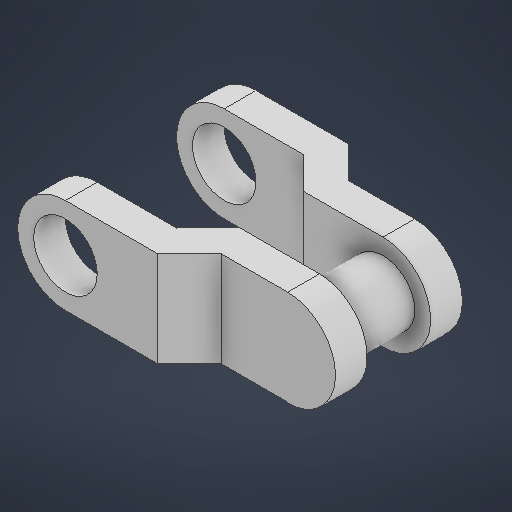
# Autodesk Inventor part: Pieza2
Saved by Autodesk Inventor 2026.2 (Build 302298010, 298A)
## iProperties
Created: 2026-03-27
Part Number: Pieza2
Material: Genérico
Document SubType Name: Modeling
Designer: agusb
Density: 1 g/cm^3
Appearance: Valor por defecto
Author: agusb
Autodesk Inventor part; units mm, degrees
ref_plane "YZ Plane" through (0, 0, 0) normal (1, 0, 0) x (0, 1, 0)
ref_plane "XZ Plane" through (0, 0, 0) normal (0, 1, 0) x (-1, 0, 0)
ref_plane "XY Plane" through (0, 0, 0) normal (0, 0, 1) x (1, 0, 0)
sketch "Boceto1" plane through (0, 0, 0) normal (0, 1, 0) x (-1, 0, 0)
  line L0 (0, -10) -> (44.14, -10)
  line L1 (44.14, -10) -> (44.14, 0)
  line L2 (44.14, 0) -> (4.14, 0)
  line L3 (4.14, 0) -> (14.14, 0) construction
  line L4 (4.14, 0) -> (14.14, 0) construction
  line L5 (-5.86, 10) -> (4.14, 0)
  line L6 (-10, 0) -> (0, -10)
  line L7 (-10, 0) -> (-45.86, 0)
  line L8 (-10, 0) -> (25.86, 0) construction
  line L9 (-45.86, 0) -> (-45.86, 10)
  line L10 (-45.86, 10) -> (-5.86, 10)
  point P0 (0, 0)
  dimension "d10" = 44.14
  dimension "d12" = 40
  dimension "d19" = 35.86
  dimension "d21" = 10
  constraints: 22 end point, 5 horizontal, 2 perpendicular, 1 collinear, 1 vertical
  measures "d10" distance of L0.start L0.end
  measures "d12" distance of L1.end L2.end
  measures "d19" distance of L6.start L7.end
  measures "d21" distance of L7.end L9.end
extrude "Extrusión1" add sketch "Boceto1" along normal blind 30
sketch "Boceto2" plane through (5.86, 0, 10) normal (0, 0, 1) x (1, 0, 0)
  point P0 (-5.86, 0)
sketch "Boceto3" plane through (0, 0, -10) normal (0, 0, -1) x (-1, 0, 0)
  line L0 (44.14, 0) -> (44.14, 30) projected
  line L1 (0, 0) -> (0, 30) projected
  line L2 (44.14, 0) -> (44.14, 15)
  line L3 (44.14, 0) -> (59.14, 0) construction
  circle A0 centre (29.14, 15) radius 10
  line L4 (0, 0) -> (44.14, 0) projected
  line L5 (29.14, 15) -> (44.14, 15) construction
  arc A1 (29.14, 0) -> (29.14, 30) centre (29.14, 15) ccw
  line L6 (44.14, 30) -> (29.14, 30)
  line L7 (44.14, 0) -> (29.14, 0)
  dimension "d24" = 44.14
  dimension "d26" = 90
  dimension "d29" = 15
  dimension "d30" = 15
  constraints: 10 end point, 3 horizontal, 3 point on circle, 2 centre point, 2 collinear, 1 perpendicular, 1 point on line, 1 tangent
  measures "d24" distance between parallel lines of L0 L1
  measures "d26" angle of L3 L2
  measures "d29" distance of L5.start L7.end
  measures "d30" distance of L5.start L6.end
extrude "Extrusión2" cut sketch "Boceto3" against normal blind 30
sketch "Boceto4" plane through (5.86, 0, 10) normal (0, 0, 1) x (1, 0, 0)
  line L0 (40, 30) -> (4.14, 30) projected
  line L1 (40, 30) -> (40, 15)
  line L2 (40, 0) -> (40, 30) projected
  circle A0 centre (25, 15) radius 7.5
  circle A1 centre (25, 15) radius 10
  arc A2 (25, 0) -> (25, 30) centre (25, 15) ccw
  line L3 (40, 0) -> (25, 0)
  point P0 (-5.86, 0)
  dimension "d34" = 15
  dimension "d37" = 15
  constraints: 4 end point, 3 centre point, 3 point on circle, 1 coincident, 1 horizontal, 1 midpoint, 1 point on line
  measures "d34" distance of L0.start L1.end
  measures "d37" diameter of A0
extrude "Extrusión3" cut sketch "Boceto4" against normal blind 30 contours L1 A2 L0 | L2 L3 A2
sketch "Boceto5" plane through (5.86, 0, 10) normal (0, 0, 1) x (1, 0, 0)
  arc A0 (25, 0) -> (25, 30) centre (25, 15) ccw projected
  line L0 (40, 15) -> (25, 15)
  circle A1 centre (25, 15) radius 10
  point P0 (-5.86, 0)
  dimension "d41" = 20
  constraints: 2 end point, 1 centre point, 1 coincident, 1 horizontal, 1 point on circle
  measures "d41" diameter of A1
extrude "Extrusión4" add sketch "Boceto5" along normal blind 20
sketch "Boceto6" plane through (30.86, 15, 30) normal (0, 0, 1) x (1, 0, 0)
  line L0 (-25, 15) -> (0, 15) projected
  arc A0 (0, -15.2696) -> (0, 15) centre (-0.1195, -0.1348) ccw
  line L1 (0, 15) -> (0, -15.2696)
  constraints: 2 end point, 2 point on circle, 1 centre point, 1 vertical
extrude "Extrusión5" add sketch "Boceto6" along normal blind 10
sketch "Boceto7" plane through (0, 30, 0) normal (0, 1, 0) x (1, 0, 0)
  line L0 (20.86, -30) -> (30.86, -30) projected
  line L1 (30.86, -30) -> (5.86, -30)
  line L2 (30.86, -30) -> (30.86, -40) projected
  line L3 (30.86, -40) -> (10, -40)
  line L4 (0, -50) -> (10, -40)
  line L5 (-4.14, -30) -> (5.86, -30) construction
  line L6 (-4.14, -40) -> (5.86, -30)
  line L7 (-4.14, -40) -> (-44.14, -40)
  line L8 (-4.14, -40) -> (35.86, -40) construction
  line L9 (-44.14, -40) -> (-44.14, -50)
  line L10 (-44.14, -50) -> (0, -50)
  point P0 (0, 0)
  dimension "d46" = 25
  dimension "d51" = 10
  dimension "d53" = 40
  dimension "d54" = 180
  dimension "d55" = 10
  dimension "d56" = 90
  constraints: 18 end point, 4 horizontal, 2 collinear, 2 perpendicular
  measures "d46" distance of L0.end L1.end
  measures "d51" distance of L5.start L6.start
  measures "d53" distance of L6.start L7.end
  measures "d54" angle of L7 L8
  measures "d55" distance of L7.end L9.end
  measures "d56" angle of L9 L7
extrude "Extrusión6" add sketch "Boceto7" against normal blind 30
sketch "Boceto8" plane through (-44.14, 30, 50) normal (0, 0, 1) x (1, 0, 0)
  line L0 (40, 0) -> (0, 0) projected
  circle A0 centre (15, -15) radius 10
  circle A1 centre (15, -15) radius 10 projected
  line L1 (0, 0) -> (0, -30) projected
  arc A2 (15, 0) -> (14.9869, -30) centre (14.9869, -15) ccw
  line L2 (0, -30) -> (40, -30) projected
  line L3 (14.9869, -30) -> (0, -30)
  point P0 (44.14, -30)
  point P1 (0, -14.3743)
  point P2 (0, -15.6257)
  dimension "d61" = 20
  constraints: 3 point on circle, 2 centre point, 2 end point, 2 point on line, 1 collinear, 1 tangent
  measures "d61" diameter of A0
extrude "Extrusión7" cut sketch "Boceto8" against normal blind 30 contours A2 L1 L0 | A2 L2 L1 | A0
